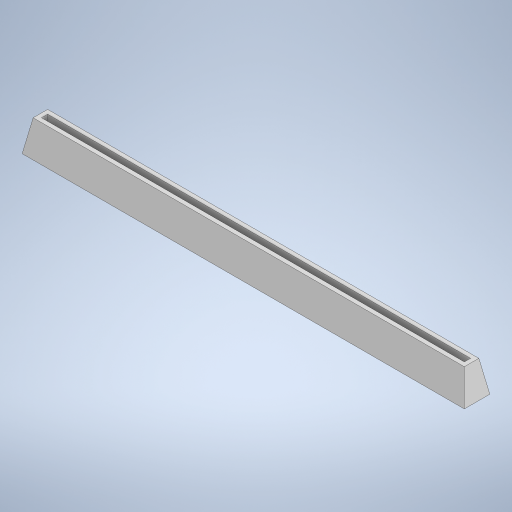
# Autodesk Inventor part: Stroemungsfilter_Fuss
Saved by Autodesk Inventor 2023 (Build 270158000, 158)
## iProperties
Created: 2023-10-04
Part Number: Stroemungsfilter_Fuss
Material: Generisch
Document SubType Name: Modeling
Designer: prigge
Density: 1 g/cm^3
Appearance: Vorgabe
Author: prigge
Autodesk Inventor part; units mm, degrees
ref_plane "YZ Plane" through (0, 0, 0) normal (1, 0, 0) x (0, 1, 0)
ref_plane "XZ Plane" through (0, 0, 0) normal (0, 1, 0) x (-1, 0, 0)
ref_plane "XY Plane" through (0, 0, 0) normal (0, 0, 1) x (1, 0, 0)
sketch "Skizze1" plane through (0, 0, 0) normal (0, 1, 0) x (-1, 0, 0)
  line L0 (102, -1.5) -> (-102, -1.5)
  line L1 (-102, -1.5) -> (-102, 1.5)
  line L2 (-102, 1.5) -> (102, 1.5)
  line L3 (102, 1.5) -> (102, -1.5)
  line L4 (104, -3.5) -> (-104, -3.5)
  line L5 (-104, -3.5) -> (-104, 3.5)
  line L6 (-104, 3.5) -> (104, 3.5)
  line L7 (104, 3.5) -> (104, -3.5)
  line L8 (0, -4.9) -> (0, 4.9) projected
  line L9 (-145.6, 0) -> (145.6, 0) projected
  point P0 (0, 0)
  dimension "d0" = 204
  dimension "d2" = 3
  dimension "d3" = 2
  dimension "d4" = 2
  constraints: 16 end point, 4 parallel, 2 horizontal, 2 perpendicular, 4 other
  measures "d0" distance between parallel lines of L1 L3
  measures "d2" distance between parallel lines of L2 L0
  measures "d3" distance between parallel lines of L4 L0
  measures "d4" distance between parallel lines of L1 L5
extrude "Extrusion1" add sketch "Skizze1" along normal blind 15 contours L3 L9 L7 L4 L8 L0 | L8 L4 L5 L9 L1 L0 | L3 L2 L8 L6 L7 L9 | L9 L5 L6 L8 L2 L1
sketch "Skizze2" plane through (0, 0, 0) normal (0, 1, 0) x (-1, 0, 0)
  line L0 (104, 3.5) -> (-104, 3.5) projected
  line L1 (104, -3.5) -> (104, 3.5) projected
  line L2 (-104, -3.5) -> (104, -3.5) projected
  line L3 (-104, 3.5) -> (-104, -3.5) projected
  point P0 (0, 0)
extrude "Extrusion2" add sketch "Skizze2" along normal blind 1
draft "Flächenverjüngung1" angle 10 pull direction (0, 1, 0) faces at (34.6667, 5, -3.5) (104, 10, 1.1667) (-34.6667, 5, 3.5) (-104, 10, -1.1667) fixed edges at (0, 15, -3.5) (104, 15, 0) (0, 15, 3.5) (-104, 15, 0)
